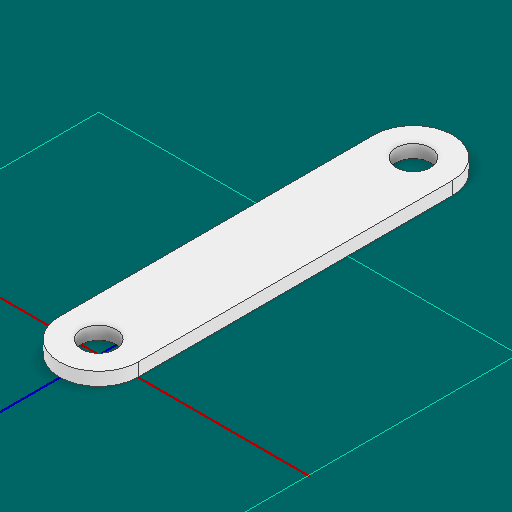
# Autodesk Inventor part: straight_gusset
Saved by Autodesk Inventor 2025 (Build 290162000, 162)
## iProperties
Created: 2024-08-16
Part Number: straight_gusset
Material: Acetal Resin, White
Document SubType Name: Modeling
Designer: averey
Density: 1.425 g/cm^3
Appearance: Smooth - White
Author: averey
Autodesk Inventor part; units mm, degrees
ref_plane "YZ Plane" through (0, 0, 0) normal (1, 0, 0) x (0, 1, 0)
ref_plane "XZ Plane" through (0, 0, 0) normal (0, 1, 0) x (-1, 0, 0)
ref_plane "XY Plane" through (0, 0, 0) normal (0, 0, 1) x (1, 0, 0)
sketch "Sketch2" plane through (0, 0, 0) normal (0, 1, 0) x (-1, 0, 0)
  circle A0 centre (0, 0) radius 2.0955
  arc A1 (-4.7625, 0) -> (-4.7625, 0) centre (0, 0) ccw
  circle A2 centre (0.0001, -38.1) radius 2.0955
  arc A3 (-4.7625, -38.1) -> (4.7628, -38.1) centre (0.0001, -38.1) ccw
  line L0 (4.7625, 0) -> (4.7628, -38.1)
  line L1 (-4.7625, 0) -> (-4.7625, -38.1)
  arc A4 (4.7625, 0) -> (-4.7625, 0) centre (0, 0) ccw
  dimension "d0" = 4.191
  dimension "d1" = 2.667
  dimension "d2" = 4.191
  dimension "d5" = 38.1
  constraints: 9 point on circle, 5 centre point, 4 end point, 3 point on line, 3 tangent, 2 coincident
  measures "d0" diameter of A0
  measures "d1" radial gap between concentric circles of A0 A1
  measures "d2" diameter of A2
  measures "d5" distance of point (0, 0) A2.centre
extrude "Extrusion1" add sketch "Sketch2" along normal blind 1.5875
body "Solid1"
